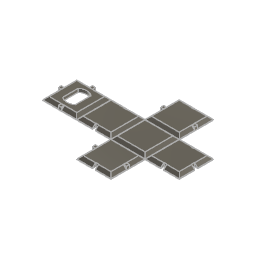
LedVoxel (Autodesk Fusion 360 design; units mm, degrees)
Autodesk Fusion 360 part; units mm, degrees
sketch "Sketch1" plane through (0, 0, 0) normal (0, 0, 1) x (1, 0, 0)
  line L0 (0, 0) -> (30, 0)
  line L1 (30, 0) -> (30, 30)
  line L2 (30, 30) -> (0, 30)
  line L3 (0, 30) -> (0, 0)
  line L4 (0, 30) -> (30, 30)
  line L5 (30, 30) -> (30, 60)
  line L6 (30, 60) -> (0, 60)
  line L7 (0, 60) -> (0, 30)
  line L8 (30, 0) -> (60, 0)
  line L9 (60, 0) -> (60, 30)
  line L10 (60, 30) -> (30, 30)
  line L11 (30, 30) -> (30, 0)
  line L12 (0, 0) -> (-30, 0)
  line L13 (-30, 0) -> (-30, 30)
  line L14 (-30, 30) -> (0, 30)
  line L15 (0, 30) -> (0, 0)
  line L16 (-30, 30) -> (-60, 30)
  line L17 (-60, 30) -> (-60, 0)
  line L18 (-60, 0) -> (-30, 0)
  line L19 (-30, 0) -> (-30, 30)
  line L20 (0, 0) -> (30, 0)
  line L21 (30, 0) -> (30, -30)
  line L22 (30, -30) -> (0, -30)
  line L23 (0, -30) -> (0, 0)
  circle A0 centre (-45, 15) radius 8.8
  line L24 (-46.3, 0) -> (-43.7, 0)
  line L25 (-43.7, 0) -> (-43.7, 2.6)
  line L26 (-43.7, 2.6) -> (-46.3, 2.6)
  line L27 (-46.3, 2.6) -> (-46.3, 0)
  line L28 (-46.3, 30) -> (-43.7, 30)
  line L29 (-43.7, 30) -> (-43.7, 27.4)
  line L30 (-43.7, 27.4) -> (-46.3, 27.4)
  line L31 (-46.3, 27.4) -> (-46.3, 30)
  line L32 (-60, 16.3) -> (-57.4, 16.3)
  line L33 (-57.4, 16.3) -> (-57.4, 13.7)
  line L34 (-57.4, 13.7) -> (-60, 13.7)
  line L35 (-60, 13.7) -> (-60, 16.3)
  line L36 (-16.3, 30) -> (-13.7, 30)
  line L37 (-13.7, 30) -> (-13.7, 26.9)
  line L38 (-13.7, 26.9) -> (-16.3, 26.9)
  line L39 (-16.3, 26.9) -> (-16.3, 30)
  line L40 (-16.3, 0) -> (-13.7, 0)
  line L41 (-13.7, 0) -> (-13.7, 3.1)
  line L42 (-13.7, 3.1) -> (-16.3, 3.1)
  line L43 (-16.3, 3.1) -> (-16.3, 0)
  line L44 (43.7, 30) -> (46.3, 30)
  line L45 (46.3, 30) -> (46.3, 26.9)
  line L46 (46.3, 26.9) -> (43.7, 26.9)
  line L47 (43.7, 26.9) -> (43.7, 30)
  line L48 (43.7, 0) -> (46.3, 0)
  line L49 (46.3, 0) -> (46.3, 3.1)
  line L50 (46.3, 3.1) -> (43.7, 3.1)
  line L51 (43.7, 3.1) -> (43.7, 0)
  line L52 (30, 46.3) -> (27.4, 46.3)
  line L53 (27.4, 46.3) -> (27.4, 43.7)
  line L54 (27.4, 43.7) -> (30, 43.7)
  line L55 (30, 43.7) -> (30, 46.3)
  line L56 (13.7, 60) -> (16.3, 60)
  line L57 (16.3, 60) -> (16.3, 56.9)
  line L58 (16.3, 56.9) -> (13.7, 56.9)
  line L59 (13.7, 56.9) -> (13.7, 60)
  line L60 (0, 46.3) -> (2.6, 46.3)
  line L61 (2.6, 46.3) -> (2.6, 43.7)
  line L62 (2.6, 43.7) -> (0, 43.7)
  line L63 (0, 43.7) -> (0, 46.3)
  line L64 (0, -13.7) -> (2.6, -13.7)
  line L65 (2.6, -13.7) -> (2.6, -16.3)
  line L66 (2.6, -16.3) -> (0, -16.3)
  line L67 (0, -16.3) -> (0, -13.7)
  line L68 (30, -13.7) -> (27.4, -13.7)
  line L69 (27.4, -13.7) -> (27.4, -16.3)
  line L70 (27.4, -16.3) -> (30, -16.3)
  line L71 (30, -16.3) -> (30, -13.7)
  line L72 (13.7, -30) -> (16.3, -30)
  line L73 (16.3, -30) -> (16.3, -26.9)
  line L74 (16.3, -26.9) -> (13.7, -26.9)
  line L75 (13.7, -26.9) -> (13.7, -30)
  line L76 (60, 16.3) -> (56.9, 16.3)
  line L77 (56.9, 16.3) -> (56.9, 13.7)
  line L78 (56.9, 13.7) -> (60, 13.7)
  line L79 (60, 13.7) -> (60, 16.3)
  line L80 (-50.6, 24.9524) -> (-39.4, 24.9524)
  line L81 (-39.4, 24.9524) -> (-39.4, 4.9524)
  line L82 (-39.4, 4.9524) -> (-50.6, 4.9524)
  line L83 (-50.6, 4.9524) -> (-50.6, 24.9524)
  line L84 (-50.6, 24.9524) -> (-39.4, 4.9524) construction
  line L85 (-50.6, 4.9524) -> (-39.4, 24.9524) construction
  point P0 (-45, 24.9524)
  dimension "d1" = 30
  dimension "d2" = 30
  dimension "d3" = 17.6
  dimension "d22" = 2.6
  dimension "d25" = 30
  dimension "d26" = 13.7
  dimension "d28" = 2.6
  dimension "d29" = 30
  dimension "d30" = 2.6
  dimension "d31" = 2.6
  dimension "d32" = 13.7
  dimension "d33" = 2.6
  dimension "d34" = 2.6
  dimension "d35" = 13.7
  dimension "d42" = 2.6
  dimension "d43" = 3.1
  dimension "d44" = 13.7
  dimension "d45" = 2.6
  dimension "d46" = 3.1
  dimension "d47" = 13.7
  dimension "d48" = 2.6
  dimension "d49" = 3.1
  dimension "d50" = 2.6
  dimension "d51" = 3.1
  dimension "d52" = 2.6
  dimension "d53" = 2.6
  dimension "d54" = 2.6
  dimension "d55" = 3.1
  dimension "d56" = 2.6
  dimension "d57" = 2.6
  dimension "d58" = 2.6
  dimension "d59" = 2.6
  dimension "d60" = 2.6
  dimension "d61" = 2.6
  dimension "d62" = 2.6
  dimension "d63" = 3.1
  dimension "d64" = 13.7
  dimension "d65" = 13.7
  dimension "d66" = 13.7
  dimension "d67" = 13.7
  dimension "d68" = 13.7
  dimension "d69" = 13.7
  dimension "d70" = 30
  dimension "d71" = 13.7
  dimension "d72" = 13.7
  dimension "d73" = 3.1
  dimension "d74" = 2.6
  dimension "d75" = 13.7
  dimension "d89" = 11.2
  dimension "d90" = 20
  dimension "d92" = 30
  dimension "d93" = 15
  dimension "d94" = 15
  constraint horizontal L0
  constraint vertical L1
  constraint horizontal L2
  constraint vertical L3
  constraint coincident L0.start L3.end
  constraint horizontal L4
  constraint vertical L5
  constraint horizontal L6
  constraint vertical L7
  constraint horizontal L8
  constraint vertical L9
  constraint horizontal L10
  constraint vertical L11
  constraint horizontal L12
  constraint vertical L13
  constraint horizontal L14
  constraint vertical L15
  constraint horizontal L16
  constraint vertical L17
  constraint vertical L19
  constraint horizontal L20
  constraint vertical L21
  constraint horizontal L22
  constraint vertical L23
  constraint horizontal L24
  constraint vertical L25
  constraint horizontal L26
  constraint vertical L27
  constraint coincident L18 L24.start
  constraint horizontal L28
  constraint vertical L29
  constraint horizontal L30
  constraint vertical L31
  constraint coincident L16 L28.start
  constraint horizontal L32
  constraint vertical L33
  constraint horizontal L34
  constraint vertical L35
  constraint coincident L17 L32.start
  constraint horizontal L36
  constraint vertical L37
  constraint horizontal L38
  constraint vertical L39
  constraint coincident L14 L36.start
  constraint horizontal L40
  constraint vertical L41
  constraint horizontal L42
  constraint vertical L43
  constraint coincident L12 L40.start
  constraint horizontal L44
  constraint vertical L45
  constraint horizontal L46
  constraint vertical L47
  constraint coincident L10 L44.start
  constraint horizontal L48
  constraint vertical L49
  constraint horizontal L50
  constraint vertical L51
  constraint coincident L8 L48.start
  constraint horizontal L52
  constraint vertical L53
  constraint horizontal L54
  constraint vertical L55
  constraint coincident L5 L52.start
  constraint horizontal L56
  constraint vertical L57
  constraint horizontal L58
  constraint vertical L59
  constraint coincident L6 L56.start
  constraint horizontal L60
  constraint vertical L61
  constraint horizontal L62
  constraint vertical L63
  constraint coincident L7 L60.start
  constraint horizontal L64
  constraint vertical L65
  constraint horizontal L66
  constraint vertical L67
  constraint coincident L23 L64.start
  constraint horizontal L68
  constraint vertical L69
  constraint horizontal L70
  constraint vertical L71
  constraint coincident L21 L68.start
  constraint horizontal L72
  constraint vertical L73
  constraint horizontal L74
  constraint vertical L75
  constraint coincident L22 L72.start
  constraint horizontal L76
  constraint vertical L77
  constraint horizontal L78
  constraint vertical L79
  constraint coincident L9 L76.start
  constraint horizontal L80
  constraint vertical L81
  constraint horizontal L82
  constraint vertical L83
  constraint midpoint L80 P0
  measures "d1" distance of L0.start L0.end
  measures "d2" distance of L0.start L2.end
  measures "d3" diameter of A0
  measures "d22" distance of L24.start L26.end
  measures "d25" distance of L17 L19
  measures "d26" distance of L17 L27
  measures "d28" distance of L25.end L26.end
  measures "d29" distance of L0.start L12.end
  measures "d30" distance of L28.start L28.end
  measures "d31" distance of L28.start L30.end
  measures "d32" distance of L17 L31
  measures "d33" distance of L32.start L32.end
  measures "d34" distance of L32.start L34.end
  measures "d35" distance of L16 L32
  measures "d42" distance of L36.start L36.end
  measures "d43" distance of L36.start L38.end
  measures "d44" distance of L13 L39
  measures "d45" distance of L40.start L40.end
  measures "d46" distance of L40.start L42.end
  measures "d47" distance of L13 L43
  measures "d48" distance of L44.start L44.end
  measures "d49" distance of L44.start L46.end
  measures "d50" distance of L48.start L48.end
  measures "d51" distance of L48.start L50.end
  measures "d52" distance of L52.start L52.end
  measures "d53" distance of L52.start L54.end
  measures "d54" distance of L56.start L56.end
  measures "d55" distance of L56.start L58.end
  measures "d56" distance of L60.start L60.end
  measures "d57" distance of L60.start L62.end
  measures "d58" distance of L64.start L64.end
  measures "d59" distance of L64.start L66.end
  measures "d60" distance of L68.start L68.end
  measures "d61" distance of L68.start L70.end
  measures "d62" distance of L72.start L72.end
  measures "d63" distance of L72.start L74.end
  measures "d64" distance of L2 L54
  measures "d65" distance of L5 L57
  measures "d66" distance of L6 L60
  measures "d67" distance of L22 L66
  measures "d68" distance of L21 L73
  measures "d69" distance of L22 L70
  measures "d70" distance of L9 L11
  measures "d71" distance of L9 L49
  measures "d72" distance of L9 L45
  measures "d73" distance of L76.start L76.end
  measures "d74" distance of L76.start L78.end
  measures "d75" distance of L10 L76
  measures "d89" distance of L80.start L80.end
  measures "d90" distance of L80.start L82.end
  measures "d92" distance of L16.end L17.end
  measures "d93" distance of L17 P0
  measures "d94" distance of L17 A0.centre
extrude "Extrude1" add sketch "Sketch1" along normal blind 3 contours L13 L16 L17 L18 L19 L25 L26 L27 L29 L30 L31 L32 L33 L34 | L18 L24 L25 L26 L27 | L16 L28 L29 L30 L31 | L17 L32 L33 L34 L35 | A0 L80 L81 L83 | A0 L81 L82 L83 makes body 1
chamfer "Chamfer1" distance 2.8 distance2 2.6 1 edges at (-45, 0, 3) measured on face at (-44.7808, 2.0749, 3) on bodies 1
chamfer "Chamfer2" distance 2.8 distance2 2.6 3 edges at (-30, 16.4, 3) (-45, 30, 3) (-60, 16.4, 3) measured on face at (-45.2192, 27.9251, 3) measured on face at (-45.2192, 27.9251, 3) measured on face at (-45.2192, 27.9251, 3) on bodies 1
extrude "Extrude2" add sketch "Sketch1" along normal blind 3 contours L3 L12 L13 L14 L15 L19 L37 L38 L39 L41 L42 L43 | L12 L40 L41 L42 L43 | L14 L36 L37 L38 L39 bodies 1
chamfer "Chamfer3" distance 2.8 distance2 2.6 4 edges at (0, 15, 3) (-15, 0, 3) (-30, 15, 3) (-15, 30, 3) measured on face at (-20, 20, 3) measured on face at (-20, 20, 3) measured on face at (-20, 20, 3) measured on face at (-20, 20, 3) on bodies 1
extrude "Extrude3" add sketch "Sketch1" along normal blind 3 contours L0 L1 L2 L3 L4 L11 L15 L20 bodies 1
chamfer "Chamfer4" distance 2.8 distance2 2.6 4 edges at (15, 30, 3) (30, 15, 3) (15, 0, 3) (0, 15, 3) measured on face at (10, 20, 3) measured on face at (10, 20, 3) measured on face at (10, 20, 3) measured on face at (10, 20, 3) on bodies 1
extrude "Extrude4" add sketch "Sketch1" along normal blind 3 contours L2 L4 L5 L6 L7 L52 L53 L54 L57 L58 L59 L60 L61 L62 | L7 L60 L61 L62 L63 | L5 L52 L53 L54 L55 | L6 L56 L57 L58 L59 bodies 1
extrude "Extrude5" add sketch "Sketch1" along normal blind 3 contours L0 L20 L21 L22 L23 L64 L65 L66 L68 L69 L70 L73 L74 L75 | L23 L64 L65 L66 L67 | L21 L68 L69 L70 L71 | L22 L72 L73 L74 L75 bodies 1
extrude "Extrude6" add sketch "Sketch1" along normal blind 3 separate body contours L1 L8 L9 L10 L11 L45 L46 L47 L49 L50 L51 L76 L77 L78 | L8 L48 L49 L50 L51 | L10 L44 L45 L46 L47 | L9 L76 L77 L78 L79 makes body 2
chamfer "Chamfer5" distance 2.8 distance2 2.6 12 edges at (30, -15, 3) (15, 0, 3) (0, -15, 3) (15, -30, 3) (15, 30, 3) (30, 45, 3) (0, 45, 3) (15, 60, 3) (45, 30, 3) (60, 15, 3) (45, 0, 3) (30, 15, 3) measured on face at (10, -10, 3) measured on face at (10, -10, 3) measured on face at (10, -10, 3) measured on face at (10, -10, 3) measured on face at (20, 40, 3) measured on face at (20, 40, 3) measured on face at (20, 40, 3) measured on face at (20, 40, 3) measured on face at (40, 20, 3) measured on face at (40, 20, 3) measured on face at (40, 20, 3) measured on face at (40, 20, 3) on bodies 1 2
extrude "Extrude7" add sketch "Sketch1" along normal blind 3 contours L16 L28 L29 L30 L31 bodies 1
extrude "Extrude8" add sketch "Sketch1" along normal blind 3 contours L17 L32 L33 L34 L35 bodies 1
extrude "Extrude9" add sketch "Sketch1" along normal blind 3 contours L18 L24 L25 L26 L27 bodies 1
extrude "Extrude10" add sketch "Sketch1" along normal blind 3 contours L23 L64 L65 L66 L67 bodies 1
extrude "Extrude11" add sketch "Sketch1" along normal blind 3 contours L21 L68 L69 L70 L71 bodies 1
extrude "Extrude12" add sketch "Sketch1" along normal blind 3 contours L7 L60 L61 L62 L63 | L5 L52 L53 L54 L55 bodies 1
extrude "Extrude13" cut sketch "Sketch1" along normal blind 3 contours L12 L40 L41 L42 L43 | L8 L48 L49 L50 L51 | L14 L36 L37 L38 L39 | L10 L44 L45 L46 L47 | L22 L72 L73 L74 L75 | L9 L76 L77 L78 L79 | L6 L56 L57 L58 L59 bodies 1 2
combine "Combine1" operation add target body 2 tool bodies 1
move_face "OffsetFaces1" offset 4.5 1 faces at (-36.2285, 14.2919, 2) on bodies 2
extrude "Extrude14" cut sketch "Sketch1" along normal blind 3 contours A0 L81 L83 bodies 2
copy_body "Body->Comp1" [suppressed] in component "Component"
copy_body "Body->Comp2" [suppressed] in component "Component'"
